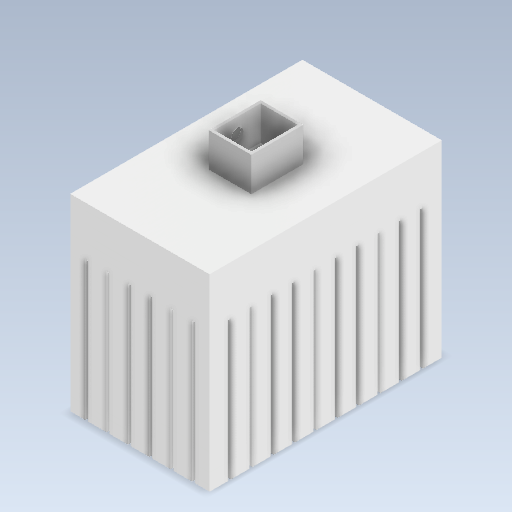
# Autodesk Inventor part: Ammonia Filter Sensor Holder
Saved by Autodesk Inventor 2020 (Build 240168000, 168)
## iProperties
Created: 2020-08-10
Part Number: Ammonia Filter Sensor Holder
Material: Generic
Document SubType Name: Modeling
Designer: Abbas
Density: 1 g/cm^3
Appearance: Default
Author: Abbas
Autodesk Inventor part; units mm, degrees
sketch "Sketch1" plane through (0, 0, 0) normal (0, 1, 0) x (-1, 0, 0)
  line L0 (75, 125) -> (-75, 125)
  line L1 (75, -122) -> (75, 125)
  line L2 (75, 125) -> (-75, 125)
  line L3 (-75, 125) -> (-75, 122)
  line L4 (-75, 122) -> (75, 122)
  line L5 (75, 122) -> (75, 125)
  line L6 (75, 125) -> (-75, 122) construction
  line L7 (-75, 125) -> (75, 122) construction
  line L8 (75, 122) -> (72, 122)
  line L9 (72, 122) -> (72, -122)
  line L10 (72, -122) -> (75, -122)
  line L11 (75, -122) -> (75, 122)
  line L12 (75, 122) -> (72, -122) construction
  line L13 (72, 122) -> (75, -122) construction
  line L14 (-72, 122) -> (-75, 122)
  line L15 (-75, 122) -> (-75, -122)
  line L16 (-75, -122) -> (-72, -122)
  line L17 (-72, -122) -> (-72, 122)
  line L18 (75, -122) -> (-75, -122)
  line L19 (-75, -122) -> (-75, -125)
  line L20 (-75, -125) -> (75, -125)
  line L21 (75, -125) -> (75, -122)
  point P0 (0, 0)
  point P1 (-75, 0)
  point P2 (0, 123.5)
  point P3 (73.5, 0)
  point P4 (75, 0)
  point P5 (72, 122)
  point P6 (-69, 125)
  point P7 (75, -122)
  point P8 (75, 122)
  point P9 (75, 122)
  point P10 (75, 122)
  dimension "d4" = 150
  dimension "d9" = 244
  dimension "d99" = 150
  dimension "d100" = 3
  constraints: 44 end point, 8 parallel, 5 horizontal, 5 midpoint, 4 perpendicular, 1 point on line
  measures "d4" distance of L4.end L3.end
  measures "d9" distance of L9.end L8.end
  measures "d99" distance of L20.end L19.end
  measures "d100" distance of L15.end L19.end
ref_plane "Work Plane8" through (0, 0, 0) normal (0, 1, 0) x (1, 0, 0)
sketch "Sketch2" plane through (0, 0, 0) normal (0, 1, 0) x (1, 0, 0)
  circle A0 centre (0, -12.655) radius 8.2
  circle A1 centre (0, 12.655) radius 8.2
  line L0 (-6.0435, -5.9922) -> (-10.65, -5.9922)
  line L1 (-10.65, -5.9922) -> (-10.65, 6.0078)
  line L2 (-10.65, 6.0078) -> (-6.0435, 6.0078)
  line L3 (-6.0435, 6.0078) -> (-6.0435, -5.9922)
  line L4 (-6.0435, -5.9922) -> (-10.65, 6.0078) construction
  line L5 (-10.65, -5.9922) -> (-6.0435, 6.0078) construction
  line L6 (0, 12.655) -> (0, -12.655)
  point P0 (0, 0)
  point P1 (0, 0)
  point P2 (-8.3467, 0.0078)
  point P3 (0, 0)
  dimension "d16" = 16.4
  dimension "d17" = 16.4
  dimension "d18" = 25.31
  dimension "d19" = 4.6065
  dimension "d20" = 12
  dimension "d21" = 12.6628
  dimension "d22" = 8.3467
  constraints: 14 end point, 3 midpoint, 2 centre point, 2 parallel, 1 coincident, 1 horizontal, 1 perpendicular, 1 vertical
  measures "d16" diameter of A0
  measures "d17" diameter of A1
  measures "d18" distance of L6.start L6.end
  measures "d19" distance of L1.end L2.end
  measures "d20" distance of L0.end L1.end
  measures "d21" vertical distance of point (-8.347, 0.008) L6.end
  measures "d22" horizontal distance of L6.end point (-8.347, 0.008)
ref_plane "Work Plane2" through (-1.5, -203, 122) normal (1, 0, 0) x (0, 0, -1)
ref_plane "Work Plane3" through (0, -203, 122) normal (1, 0, 0) x (0, 0, -1)
extrude "Extrusion10" add sketch "Sketch1" against normal blind 3 contours L9 L18 L17 L4
extrude "Extrusion11" add sketch "Sketch1" against normal blind 203 contours L1 L4 L3 L0 | L1 L10 L9 L4 | L4 L17 L16 L15 | L21 L20 L19 L16 L18 L10
extrude "Extrusion12" cut sketch "Sketch2" against normal blind 3
ref_plane "Work Plane9" through (0, -203, 122) normal (1, 0, 0) x (0, 0, -1)
sketch "Sketch10" plane through (0, -203, 122) normal (1, 0, 0) x (0, 0, -1)
  line L0 (117.545, 203) -> (117.545, 200) projected
  line L1 (142.855, 200) -> (126.455, 200) projected
  line L2 (117.545, 200) -> (126.455, 200)
  line L3 (117.545, 200) -> (126.455, 200) construction
  line L4 (122, 200.3003) -> (122, 0.3003)
  line L5 (122, 200.3003) -> (322, 200.3003) construction
  line L6 (122, 199.5774) -> (22, 26.3723)
  line L7 (122, 199.5774) -> (322, 199.5774) construction
  line L8 (122, 200.3003) -> (222, 27.0952)
  line L9 (122, 200.3003) -> (322, 200.3003) construction
  point P0 (122, 203)
  dimension "d110" = 0
  dimension "d111" = 200
  dimension "d112" = 90
  dimension "d113" = 200
  dimension "d114" = 120
  dimension "d115" = 200
  dimension "d116" = 60
  constraints: 16 end point, 5 horizontal, 4 equal length, 2 point on line, 1 vertical
  measures "d110" distance between parallel lines of L2 L3
  measures "d111" distance of L4.start L4.end
  measures "d112" angle of L4 L5
  measures "d113" distance of L6.start L6.end
  measures "d114" angle of L6 L7
  measures "d115" distance of L4.start L8.end
  measures "d116" angle of L8 L9
sketch "Sketch12" plane through (-75, 0, 125) normal (0, 0, 1) x (1, 0, 0)
  line L0 (16, -53) -> (19, -53)
  line L1 (19, -53) -> (19, -203)
  line L2 (19, -203) -> (16, -203)
  line L3 (16, -203) -> (16, -53)
  line L4 (16, -53) -> (19, -203) construction
  line L5 (19, -53) -> (16, -203) construction
  line L6 (150, -203) -> (0, -203) projected
  line L7 (0, 0) -> (0, -203) projected
  line L8 (39, -53) -> (42, -53)
  line L9 (39, -203) -> (39, -53)
  line L10 (39, -53) -> (42, -203) construction
  line L11 (42, -53) -> (39, -203) construction
  line L12 (42, -53) -> (42, -203)
  line L13 (42, -203) -> (39, -203)
  line L14 (62, -53) -> (65, -53)
  line L15 (62, -203) -> (62, -53)
  line L16 (62, -53) -> (65, -203) construction
  line L17 (65, -53) -> (62, -203) construction
  line L18 (65, -53) -> (65, -203)
  line L19 (65, -203) -> (62, -203)
  line L20 (85, -53) -> (88, -53)
  line L21 (85, -203) -> (85, -53)
  line L22 (85, -53) -> (88, -203) construction
  line L23 (88, -53) -> (85, -203) construction
  line L24 (88, -53) -> (88, -203)
  line L25 (88, -203) -> (85, -203)
  line L26 (108, -53) -> (111, -53)
  line L27 (108, -203) -> (108, -53)
  line L28 (108, -53) -> (111, -203) construction
  line L29 (111, -53) -> (108, -203) construction
  line L30 (111, -53) -> (111, -203)
  line L31 (111, -203) -> (108, -203)
  line L32 (131, -53) -> (134, -53)
  line L33 (131, -203) -> (131, -53)
  line L34 (131, -53) -> (134, -203) construction
  line L35 (134, -53) -> (131, -203) construction
  line L36 (134, -53) -> (134, -203)
  line L37 (134, -203) -> (131, -203)
  point P0 (75, 0)
  point P1 (17.5, -128)
  point P2 (17.5, -203)
  point P3 (40.5, -128)
  point P4 (40.5, -203)
  point P5 (63.5, -128)
  point P6 (63.5, -203)
  point P7 (86.5, -128)
  point P8 (86.5, -203)
  point P9 (109.5, -128)
  point P10 (109.5, -203)
  point P11 (132.5, -128)
  point P12 (132.5, -203)
  dimension "d119" = 3
  dimension "d120" = 150
  dimension "d121" = 16
  dimension "d124" = 23
  constraints: 72 end point, 13 midpoint, 2 horizontal, 2 parallel, 1 perpendicular, 1 point on line, 60 other
  measures "d119" distance of L1.end L2.end
  measures "d120" distance of L0.end L1.end
  measures "d121" distance between parallel lines of L7 L3
  measures "d124" distance of L0.start L8.start
extrude "Extrusion13" cut sketch "Sketch12" against normal blind 300
sketch "Sketch13" plane through (-75, 0, -125) normal (-1, 0, 0) x (0, 0, 1)
  line L0 (20, -53) -> (23, -53)
  line L1 (23, -53) -> (23, -203)
  line L2 (23, -203) -> (20, -203)
  line L3 (20, -203) -> (20, -53)
  line L4 (20, -53) -> (23, -203) construction
  line L5 (23, -53) -> (20, -203) construction
  line L6 (250, -203) -> (0, -203) projected
  line L7 (0, 0) -> (0, -203) projected
  line L8 (43, -53) -> (46, -53)
  line L9 (46, -53) -> (46, -203)
  line L10 (43, -203) -> (43, -53)
  line L11 (43, -53) -> (46, -203) construction
  line L12 (46, -53) -> (43, -203) construction
  line L13 (46, -203) -> (43, -203)
  line L14 (66, -53) -> (69, -53)
  line L15 (69, -53) -> (69, -203)
  line L16 (66, -203) -> (66, -53)
  line L17 (66, -53) -> (69, -203) construction
  line L18 (69, -53) -> (66, -203) construction
  line L19 (69, -203) -> (66, -203)
  line L20 (89, -53) -> (92, -53)
  line L21 (92, -53) -> (92, -203)
  line L22 (89, -203) -> (89, -53)
  line L23 (89, -53) -> (92, -203) construction
  line L24 (92, -53) -> (89, -203) construction
  line L25 (92, -203) -> (89, -203)
  line L26 (112, -53) -> (115, -53)
  line L27 (115, -53) -> (115, -203)
  line L28 (112, -203) -> (112, -53)
  line L29 (112, -53) -> (115, -203) construction
  line L30 (115, -53) -> (112, -203) construction
  line L31 (115, -203) -> (112, -203)
  line L32 (135, -53) -> (138, -53)
  line L33 (138, -53) -> (138, -203)
  line L34 (135, -203) -> (135, -53)
  line L35 (135, -53) -> (138, -203) construction
  line L36 (138, -53) -> (135, -203) construction
  line L37 (138, -203) -> (135, -203)
  line L38 (158, -53) -> (161, -53)
  line L39 (161, -53) -> (161, -203)
  line L40 (158, -203) -> (158, -53)
  line L41 (158, -53) -> (161, -203) construction
  line L42 (161, -53) -> (158, -203) construction
  line L43 (161, -203) -> (158, -203)
  line L44 (181, -53) -> (184, -53)
  line L45 (184, -53) -> (184, -203)
  line L46 (181, -203) -> (181, -53)
  line L47 (181, -53) -> (184, -203) construction
  line L48 (184, -53) -> (181, -203) construction
  line L49 (184, -203) -> (181, -203)
  line L50 (204, -53) -> (207, -53)
  line L51 (207, -53) -> (207, -203)
  line L52 (204, -203) -> (204, -53)
  line L53 (204, -53) -> (207, -203) construction
  line L54 (207, -53) -> (204, -203) construction
  line L55 (207, -203) -> (204, -203)
  line L56 (227, -53) -> (230, -53)
  line L57 (230, -53) -> (230, -203)
  line L58 (227, -203) -> (227, -53)
  line L59 (227, -53) -> (230, -203) construction
  line L60 (230, -53) -> (227, -203) construction
  line L61 (230, -203) -> (227, -203)
  point P0 (125, 0)
  point P1 (21.5, -128)
  point P2 (21.5, -203)
  point P3 (44.5, -128)
  point P4 (44.5, -203)
  point P5 (67.5, -128)
  point P6 (67.5, -203)
  point P7 (90.5, -128)
  point P8 (90.5, -203)
  point P9 (113.5, -128)
  point P10 (113.5, -203)
  point P11 (136.5, -128)
  point P12 (136.5, -203)
  point P13 (159.5, -128)
  point P14 (159.5, -203)
  point P15 (182.5, -128)
  point P16 (182.5, -203)
  point P17 (205.5, -128)
  point P18 (205.5, -203)
  point P19 (228.5, -128)
  point P20 (228.5, -203)
  dimension "d131" = 3
  dimension "d132" = 150
  dimension "d133" = 20
  dimension "d136" = 23
  constraints: 120 end point, 21 midpoint, 2 horizontal, 2 parallel, 1 perpendicular, 1 point on line, 108 other
  measures "d131" distance of L1.end L2.end
  measures "d132" distance of L0.end L1.end
  measures "d133" distance between parallel lines of L7 L3
  measures "d136" distance of L0.start L8.start
extrude "Extrusion14" cut sketch "Sketch13" against normal blind 200
sketch "Sketch14" plane through (0, 0, 0) normal (0, 1, 0) x (1, 0, 0)
  line L0 (-20, -25) -> (20, -25)
  line L1 (20, -28) -> (20, 28)
  line L2 (20, 25) -> (-20, 25)
  line L3 (-20, 28) -> (-20, -28)
  line L4 (-23, -28) -> (23, -28)
  line L5 (23, -28) -> (23, 28)
  line L6 (23, 28) -> (-23, 28)
  line L7 (-23, 28) -> (-23, -28)
  point P0 (0, 0)
  constraints: 16 end point, 8 point on line, 4 parallel, 2 horizontal, 2 perpendicular
extrude "Extrusion15" add sketch "Sketch14" along normal blind 37 contours L3 L4 L7 L6 | L0 L1 L4 L3 | L1 L6 L5 L4 | L3 L6 L1 L2
sketch "Sketch16" plane through (-23, 0, -28) normal (-1, 0, 0) x (0, 0, 1)
  circle A0 centre (28, 20) radius 6.5
  point P0 (28, 0)
  dimension "d153" = 13
  constraints: 1 centre point
  measures "d153" diameter of A0
extrude "Extrusion17" cut sketch "Sketch16" against normal blind 10
body "Solid2"
